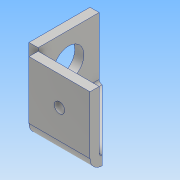
# Autodesk Inventor part: Top_Cable End
Saved by Autodesk Inventor 2018.1 (Build 221171000, 171)
## iProperties
Created: 2019-03-23
Part Number: Top_Cable End
Material: Aluminum 6061
Document SubType Name: Modeling
Designer: James
Density: 2.7 g/cm^3
Appearance: Aluminum - Flat
Author: James
Autodesk Inventor part; units mm, degrees
ref_plane "YZ Plane" through (0, 0, 0) normal (1, 0, 0) x (0, 1, 0)
ref_plane "XZ Plane" through (0, 0, 0) normal (0, 1, 0) x (-1, 0, 0)
ref_plane "XY Plane" through (0, 0, 0) normal (0, 0, 1) x (1, 0, 0)
sketch "Sketch1" plane through (0, 0, 0) normal (0, 0, 1) x (1, 0, 0)
  line L0 (0, 0) -> (24, 0)
  line L1 (24, 0) -> (24, 24)
  line L2 (24, 24) -> (0, 24)
  line L3 (0, 24) -> (0, 0)
  line L4 (4, 24) -> (24, 4)
  dimension "d0" = 45
  dimension "d1" = 24
  dimension "d2" = 24
  dimension "d3" = 4
  constraints: 10 end point, 2 parallel, 2 point on line, 1 horizontal, 1 perpendicular
  measures "d0" angle of L2 L4
  measures "d1" distance of L2.end L0.start
  measures "d2" distance of L0.start L0.end
  measures "d3" distance from line of L4.start L3
extrude "Extrusion1" add sketch "Sketch1" along normal blind 3 contours L3 L2 L4 L1 L0
sketch "Sketch2" plane through (0, 0, 3) normal (0, 0, 1) x (1, 0, 0)
  line L0 (0, 0) -> (24, 0) projected
  line L1 (24, 0) -> (24, 4) projected
  line L2 (24, 4) -> (4, 24) projected
  line L3 (4, 24) -> (0, 24) projected
  line L4 (0, 24) -> (0, 0) projected
  line L5 (4, 24) -> (0, 24) projected
  line L6 (0, 0) -> (3, 0)
  line L7 (3, 0) -> (3, 24)
  line L8 (3, 24) -> (0, 24)
  line L9 (0, 24) -> (0, 0)
  line L10 (24, 3) -> (0, 3)
  line L11 (0, 3) -> (0, 0)
  line L12 (0, 0) -> (24, 0)
  line L13 (24, 0) -> (24, 3)
  dimension "d20" = 3
  dimension "d21" = 3
  constraints: 16 end point, 4 parallel, 2 horizontal, 2 perpendicular, 2 point on line
  measures "d20" distance between parallel lines of L4 L7
  measures "d21" distance between parallel lines of L0 L10
extrude "Extrusion2" add sketch "Sketch2" along normal blind 20 contours L4 L10 L7 L0 | L7 L10 L1 L0 | L4 L3 L7 L10
sketch "Sketch6" plane through (0, 0, 23) normal (0, 0, 1) x (1, 0, 0)
  line L0 (0, 0) -> (4, 0)
  line L1 (4, 0) -> (4, 4)
  line L2 (4, 4) -> (0, 4)
  line L3 (0, 4) -> (0, 0)
  line L4 (3, 3) -> (3, 24) projected
  line L5 (24, 3) -> (3, 3) projected
  dimension "d22" = 1
  dimension "d23" = 1
  constraints: 8 end point, 2 parallel, 1 horizontal, 1 perpendicular
  measures "d22" distance between parallel lines of L1 L4
  measures "d23" distance between parallel lines of L2 L5
extrude "Extrusion5" cut sketch "Sketch6" against normal through all
fillet "Fillet1" radius 1 2 edges at (3, 14, 3) (14, 3, 3)
fillet "Fillet2" radius 4 2 edges at (0, 14, 0) (14, 0, 0)
sketch "Sketch7" plane through (3, 4, 23) normal (1, 0, 0) x (0, 0, -1)
  line L0 (0, 0) -> (0, 20) projected
  line L1 (19, 20) -> (0, 20) projected
  point P0 (23, -4)
  point P1 (9.5, 10)
  point P2 (0, 10)
  point P3 (9.5, 20)
  constraints: 2 midpoint, 1 horizontal alignment, 1 vertical alignment
hole "Hole1" at (3, 14, 13.5) direction (-1, 0, 0) diameter 10 end through all
sketch "Sketch8" plane through (4, 3, 23) normal (0, 1, 0) x (1, 0, 0)
  line L0 (0, 19) -> (0, 0) projected
  line L1 (20, 0) -> (0, 0) projected
  point P0 (-4, 23)
  point P1 (10, 9.5)
  point P2 (0, 9.5)
  point P3 (10, 0)
  constraints: 2 midpoint, 1 horizontal alignment, 1 vertical alignment
hole "Hole2" at (14, 3, 13.5) direction (0, -1, 0) diameter 3.4 end through all clearance for "Flat Head Machine Screw" size "M3" standard "Ansi Metric M Profile"
equation "\"d2\" = d1"
equation "\"d21\" = d20"
equation "\"d23\" = d22"
body "Solid1"
